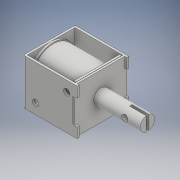
# Autodesk Inventor part: Соленоид
Saved by Autodesk Inventor 2017 (Build 210142000, 142)
## iProperties
Part Number: Соленоид
Material: Типовые
Document SubType Name: Modeling
Designer: Daemon
Density: 1 g/cm^3
Appearance: По умолчанию
Author: Daemon
Autodesk Inventor part; units mm, degrees
note: some values were not read from the file. Chosen so that the rebuilt part matches the saved one: copy form of "Зеркальное отражение4".
sketch "Эскиз1" plane through (0, 0, 0) normal (0, 0, 1) x (1, 0, 0)
  line L0 (0, 0) -> (0, 25)
  line L1 (0, 25) -> (26, 25)
  line L2 (26, 25) -> (26, 0)
  line L3 (26, 0) -> (0, 0)
  dimension "d2" = 25
  dimension "d3" = 26
  constraints: 8 end point, 3 perpendicular, 1 vertical
  measures "d2" distance of L0.start L0.end
  measures "d3" distance of L0.end L1.end
extrude "Выдавливание1" add sketch "Эскиз1" against normal blind 22
sketch "Эскиз4" plane through (0, 0, 0) normal (0, 0, 1) x (1, 0, 0)
  line L0 (1, 1) -> (26, 1)
  line L1 (26, 25) -> (26, 0) projected
  line L2 (1, 1) -> (1, 24)
  line L3 (1, 24) -> (26, 24)
  line L4 (26, 1) -> (26, 24)
  line L5 (0, 25) -> (26, 25) projected
  line L6 (26, 0) -> (0, 0) projected
  line L7 (0, 0) -> (0, 25) projected
  dimension "d16" = 1
  dimension "d17" = 1
  dimension "d18" = 1
  constraints: 8 end point, 2 point on line, 1 collinear, 1 horizontal, 1 perpendicular, 1 vertical
  measures "d16" distance from line of L5 L2.end
  measures "d17" distance from line of L6 L0.start
  measures "d18" distance from line of L7 L2.end
extrude "Выдавливание4" cut sketch "Эскиз4" against normal through all contours L2 L3 L1 L0
sketch "Эскиз5" plane through (0, 0, 0) normal (0, -1, 0) x (1, 0, 0)
  line L0 (26, 0) -> (26, -22) projected
  line L1 (26, -5) -> (24, -5)
  line L2 (26, -17) -> (24, -17)
  line L3 (24, -17) -> (24, -5)
  line L4 (26, 0) -> (0, 0) projected
  line L5 (26, -5) -> (26, -17)
  dimension "d21" = 5
  dimension "d22" = 5
  dimension "d23" = 2
  constraints: 8 end point, 2 horizontal, 2 point on line, 1 collinear, 1 perpendicular
  measures "d21" distance from line of L4 L1.start
  measures "d22" distance of L0.end L2.start
  measures "d23" distance of L1.start L1.end
extrude "Выдавливание5" cut sketch "Эскиз5" against normal through all
sketch "Эскиз6" plane through (1, 1, 0) normal (1, 0, 0) x (0, 0, -1)
  line L0 (0, 0) -> (0, -1) projected
  line L1 (22, 24) -> (22, 23) projected
  line L2 (22, 0) -> (22, -1) projected
  line L3 (0, 23) -> (5, 23) projected
  circle A0 centre (11, 11.5) radius 11
  line L4 (0, -1) -> (0, 24) projected
  dimension "d26" = 22
  constraints: 1 centre point, 1 tangent
  measures "d26" diameter of A0
extrude "Выдавливание6" add sketch "Эскиз6" along normal blind 1
sketch "Эскиз7" plane through (2, 12.5, -11) normal (1, 0, 0) x (0, 0, -1)
  circle A0 centre (0, 0) radius 10.5
  point P0 (-11, -12.5)
  dimension "d29" = 21
  constraints: 1 centre point
  measures "d29" diameter of A0
extrude "Выдавливание7" add sketch "Эскиз7" along normal blind 21
sketch "Эскиз8" plane through (23, 12.5, -11) normal (1, 0, 0) x (0, 0, -1)
  line L0 (-6, -11.5) -> (-11, -11.5) projected
  line L1 (-11, 12.5) -> (-11, 11.5) projected
  line L2 (6, 11.5) -> (11, 11.5) projected
  line L3 (11, -12.5) -> (11, 12.5) projected
  line L4 (-11, -11.5) -> (-11, -12.5) projected
  line L5 (11, -11.5) -> (6, -11.5) projected
  line L6 (0, -11) -> (-11, -11)
  line L7 (0, -11) -> (11, -11)
  line L8 (0, 11) -> (-11, 11)
  line L9 (-11, -12.5) -> (-11, 12.5) projected
  line L10 (0, 11) -> (11, 11)
  line L11 (11, -11) -> (11, 11)
  line L12 (-11, -11) -> (-11, 11)
  point P0 (11, 0)
  point P1 (-11, 0)
  constraints: 12 end point, 4 point on line, 2 collinear, 2 horizontal, 2 perpendicular
extrude "Выдавливание8" add sketch "Эскиз8" along normal blind 1
ref_plane "РабПлоскость1" through (25, 12.5, -11) normal (1, 0, 0) x (0, 0, -1)
sketch "Эскиз13" plane through (25, 12.5, -11) normal (1, 0, 0) x (0, 0, -1)
  line L0 (-6, -12.5) -> (-6, -11.5) projected
  line L1 (-6, -11.5) -> (-6, -12.5)
  line L2 (6, -11.5) -> (6, -12.5) projected
  line L3 (-6, -12.5) -> (6, -12.5)
  line L4 (6, -12.5) -> (6, -11.5)
  line L5 (6, -11.5) -> (11, -11.5)
  line L6 (6, 11.5) -> (11, 11.5) projected
  line L7 (11, -11.5) -> (11, 11.5)
  line L8 (11, 11.5) -> (6, 11.5)
  line L9 (6, 11.5) -> (6, 12.5)
  line L10 (-6, 12.5) -> (6, 12.5) projected
  line L11 (6, 12.5) -> (-6, 12.5)
  line L12 (-6, 11.5) -> (-6, 12.5) projected
  line L13 (-6, 12.5) -> (-6, 11.5)
  line L14 (-11, 11.5) -> (-6, 11.5) projected
  line L15 (-6, 11.5) -> (-11, 11.5)
  line L16 (-6, -11.5) -> (-11, -11.5) projected
  line L17 (-11, 11.5) -> (-11, -11.5)
  line L18 (-11, -11.5) -> (-6, -11.5)
  line L19 (-11, -11) -> (11, -11) projected
  point P0 (-11, -12.5)
  constraints: 24 end point, 9 perpendicular, 1 collinear, 1 parallel, 1 vertical
extrude "Выдавливание11" add sketch "Эскиз13" against normal blind 0.9
ref_plane "РабПлоскость2" through (0, 12.5, 0) normal (0, -1, 0) x (1, 0, 0)
sketch "Эскиз14" plane through (0, 0, 0) normal (0, -1, 0) x (1, 0, 0)
  circle A0 centre (6, -17) radius 1.5
  line L0 (0, 0) -> (0, -22) projected
  line L1 (26, -22) -> (0, -22) projected
  dimension "d42" = 6
  dimension "d43" = 5
  dimension "d44" = 3
  constraints: 1 centre point
  measures "d42" distance from line of L0 A0.centre
  measures "d43" distance from line of L1 A0.centre
  measures "d44" diameter of A0
extrude "Выдавливание12" cut sketch "Эскиз14" against normal blind 1
sketch "Эскиз15" plane through (0, 0, 0) normal (0, -1, 0) x (1, 0, 0)
  circle A0 centre (21, -5) radius 1.5
  line L0 (0, 0) -> (0, -22) projected
  line L1 (26, 0) -> (0, 0) projected
  dimension "d47" = 3
  dimension "d48" = 21
  dimension "d49" = 5
  constraints: 1 centre point
  measures "d47" diameter of A0
  measures "d48" distance from line of L0 A0.centre
  measures "d49" distance from line of L1 A0.centre
extrude "Выдавливание13" cut sketch "Эскиз15" against normal blind 1
mirror "Зеркальное отражение1" about plane through (0, 12.5, 0) normal (0, -1, 0) of "Выдавливание12"
mirror "Зеркальное отражение2" about plane through (0, 12.5, 0) normal (0, -1, 0) of "Выдавливание13"
sketch "Эскиз16" plane through (25, 12.5, -11) normal (1, 0, 0) x (0, 0, -1)
  circle A0 centre (0, 0) radius 3.5
  point P0 (-11, -12.5)
  dimension "d52" = 7
  constraints: 1 centre point
  measures "d52" diameter of A0
extrude "Выдавливание14" add sketch "Эскиз16" along normal blind 22.5
ref_plane "РабПлоскость3" through (25, 12.5, -7.5) normal (0, 0, 1) x (1, 0, 0)
sketch "Эскиз17" plane through (25, 12.5, -7.5) normal (0, 0, 1) x (1, 0, 0)
  line L0 (22.5, -3.5) -> (22.5, 3.5) projected
  line L1 (22.5, 0) -> (14.5, 0)
  line L2 (14.5, 0) -> (14.5, 0.625)
  line L3 (14.5, 0.625) -> (22.5, 0.625)
  line L4 (22.5, 0) -> (22.5, 0.625)
  point P0 (-25, -12.5)
  dimension "d55" = 1.25
  dimension "d56" = 8
  constraints: 8 end point, 1 collinear, 1 horizontal, 1 midpoint, 1 perpendicular, 1 point on line, 1 vertical
  measures "d55" diameter of L3 L1
  measures "d56" distance of L2.end L3.end
extrude "Выдавливание15" cut sketch "Эскиз17" against normal through all
mirror "Зеркальное отражение3" about plane through (47.5, 12.5, -7.5) normal (0, 1, 0) of "Выдавливание15"
fillet "Сопряжение1" radius 1 1 edges at (0, 0, -11)
fillet "Сопряжение2" radius 1 1 edges at (0, 25, -11)
ref_plane "РабПлоскость4" through (25, 9, -11) normal (0, 1, 0) x (-1, 0, 0)
sketch "Эскиз18" plane through (25, 9, -11) normal (0, 1, 0) x (-1, 0, 0)
  line L0 (0, 3.5) -> (-14.5, 3.5) projected
  line L1 (0, -3.5) -> (-14.5, -3.5) projected
  circle A0 centre (-15, 0) radius 1.5
  line L2 (25, 11) -> (25, -11) projected
  dimension "d63" = 3
  dimension "d64" = 40
  constraints: 1 centre point
  measures "d63" diameter of A0
  measures "d64" distance from line of L2 A0.centre
extrude "Выдавливание16" cut sketch "Эскиз18" along normal up to next
mirror "Зеркальное отражение4" about plane through (0, 12.5, 0) normal (0, -1, 0) of "Выдавливание16" geometry pattern yes
sketch "Эскиз19" plane through (0, 1, -22) normal (-1, 0, 0) x (0, 0, 1)
  line L0 (22, 24) -> (22, 23) projected
  line L1 (0, 0) -> (0, -1) projected
  line L2 (0, 24) -> (0, 23) projected
  line L3 (22, 0) -> (17, 0) projected
  circle A0 centre (11, 11.5) radius 2.5
  point P0 (22, -1)
  dimension "d67" = 5
  constraints: 1 centre point
  measures "d67" diameter of A0
extrude "Выдавливание17" add sketch "Эскиз19" along normal blind 2
fillet "Сопряжение5" radius 0.5 1 edges at (-2, 12.5, -13.5)
sketch "Эскиз20" plane through (-2, 12.5, -11) normal (-1, 0, 0) x (0, 0, 1)
  circle A0 centre (0, 0) radius 2.5 projected
  line L0 (2.1651, 1.25) -> (2.1651, -1.25)
  line L1 (0, -2.5) -> (2.1651, -1.25)
  line L2 (2.1651, 1.25) -> (0, 2.5)
  line L3 (-2.1651, 1.25) -> (-2.1651, -1.25)
  line L4 (0, -2.5) -> (-2.1651, -1.25)
  line L5 (-2.1651, 1.25) -> (0, 2.5)
  point P0 (11, -12.5)
  dimension "d73" = 120
  dimension "d74" = 120
  dimension "d75" = 4.3301
  dimension "d76" = 8.8349
  dimension "d77" = 7.4904
  constraints: 12 end point, 5 equal length, 1 parallel, 1 vertical
  measures "d73" angle of L2 L0
  measures "d74" angle of L1 L0
  measures "d75" distance between parallel lines of L1 L5
  measures "d76" distance from line of point (11, -12.5) L0
  measures "d77" distance from line of point (11, -12.5) L2
extrude "Выдавливание18" add sketch "Эскиз20" along normal blind 6 contours L0 L1 L4 L3 L5 L2
